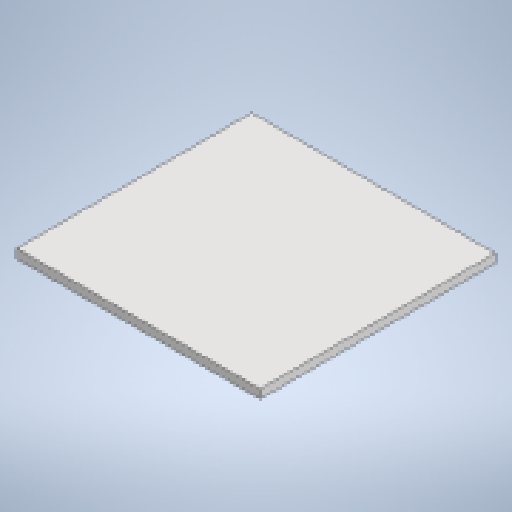
# Autodesk Inventor part: PLACA BASE
Saved by Autodesk Inventor 2024.1 (Build 281209000, 209)
## iProperties
Created: 2025-06-24
Part Number: PLACA BASE
Material: Generic
Document SubType Name: Modeling
Designer: User
Density: 1 g/cm^3
Appearance: Default
Author: User
Autodesk Inventor part; units mm, degrees
ref_plane "YZ Plane" through (0, 0, 0) normal (1, 0, 0) x (0, 1, 0)
ref_plane "XZ Plane" through (0, 0, 0) normal (0, 1, 0) x (-1, 0, 0)
ref_plane "XY Plane" through (0, 0, 0) normal (0, 0, 1) x (1, 0, 0)
sketch "Sketch1" plane through (0, 0, 0) normal (0, 1, 0) x (-1, 0, 0)
  line L0 (-175, -169) -> (175, -169)
  line L1 (175, -169) -> (175, 169)
  line L2 (175, 169) -> (-175, 169)
  line L3 (-175, 169) -> (-175, -169)
  line L4 (-175, -169) -> (175, 169) construction
  line L5 (175, -169) -> (-175, 169) construction
  point P0 (0, 0)
  dimension "d0" = 338
  dimension "d1" = 350
  constraints: 12 end point, 2 midpoint, 2 parallel, 1 horizontal, 1 perpendicular
  measures "d0" distance of L2.end L0.start
  measures "d1" distance of L1.end L2.end
extrude "Extrusion1" add sketch "Sketch1" along normal blind 12.7
sketch "Sketch2" plane through (0, 0, 0) normal (0, -1, 0) x (1, 0, 0)
  circle A0 centre (-97.564, 92.95) radius 12 projected
  circle A1 centre (-97.564, -15.05) radius 12 projected
  circle A2 centre (-97.564, -15.05) radius 12 projected
  circle A3 centre (100.436, 92.95) radius 12 projected
  circle A4 centre (100.436, -15.05) radius 12 projected
  circle A5 centre (-125.564, 127) radius 6.73 projected
  circle A6 centre (-125.564, 82.6) radius 6.73 projected
  circle A7 centre (-125.564, -82.6) radius 6.73 projected
  circle A8 centre (-125.564, -127) radius 6.73 projected
  circle A9 centre (128.436, -127) radius 6.73 projected
  circle A10 centre (128.436, -82.6) radius 6.73 projected
  circle A11 centre (128.436, 82.6) radius 6.73 projected
  circle A12 centre (128.436, 127) radius 6.73 projected
  point P0 (0, 0)
extrude "Extrusion2" cut sketch "Sketch2" against normal blind 10
sketch "Sketch3" plane through (0, 0, 0) normal (0, -1, 0) x (1, 0, 0)
  circle A0 centre (-97.564, -15.05) radius 12 projected
  circle A1 centre (-97.564, 92.95) radius 12 projected
  circle A2 centre (100.436, -15.05) radius 12 projected
  circle A3 centre (100.436, 92.95) radius 12 projected
  point P0 (0, 0)
  constraints: 4 coincident
hole "Hole1" at (-97.564, 0, -15.05) at (-97.564, 0, 92.95) at (100.436, 0, -15.05) at (100.436, 0, 92.95) direction (0, 1, 0) diameter 26.211 depth 12.7 thread size "M30x3.5" class "6H" standard "ANSI Metric M Profile"
body "Solid1"
